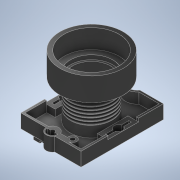
# Autodesk Inventor part: BASE DO BOTÃO
Saved by Autodesk Inventor 2022 (Build 260153000, 153)
## iProperties
Created: 2023-07-19
Part Number: BASE DO BOTÃO
Material: Acetal Resin, Black
Document SubType Name: Modeling
Designer: Usuário
Density: 1.425 g/cm^3
Appearance: Glossy - Black
Author: Usuário
Autodesk Inventor part; units mm, degrees
sketch "Sketch1" plane through (0, 0, 0) normal (0, 1, 0) x (-1, 0, 0)
  line L0 (0, 0) -> (30, 0)
  line L1 (30, 0) -> (30, -40)
  line L2 (30, -40) -> (0, -40)
  line L3 (0, -40) -> (0, 0)
  dimension "d0" = 30
  dimension "d1" = 40
  constraints: 8 end point, 2 parallel, 1 horizontal, 1 perpendicular
  measures "d0" distance of L1.end L2.end
  measures "d1" distance of L0.end L1.end
extrude "Extrusion1" add sketch "Sketch1" along normal blind 6.5
sketch "Sketch2" plane through (0, 0, 0) normal (0, -1, 0) x (1, 0, 0)
  circle A0 centre (-15, -20) radius 9
  line L0 (0, 0) -> (0, -40) projected
  line L1 (0, -40) -> (-30, -40) projected
  line L2 (0, 0) -> (0, -40) projected
  line L3 (0, -20) -> (-30, -20) construction
  line L4 (-30, -40) -> (-30, 0) projected
  line L5 (0, -40) -> (-30, -40) projected
  line L6 (-2.3, -14.5) -> (-2.3, -25.5) construction
  line L7 (-1.7, -14.5) -> (-2.9, -14.5)
  line L8 (-1.7, -25.5) -> (-2.9, -25.5)
  line L9 (-1.7, -14.5) -> (-1.7, -18.0921)
  line L10 (-1.7, -21.9079) -> (-1.7, -25.5)
  arc A1 (-2.9, -18.0921) -> (-2.9, -21.9079) centre (-2.3, -20) ccw
  arc A2 (-1.7, -21.9079) -> (-1.7, -18.0921) centre (-2.3, -20) ccw
  line L11 (-2.9, -14.5) -> (-2.9, -18.0921)
  line L12 (-2.9, -21.9079) -> (-2.9, -25.5)
  line L13 (-27.7, -14.5) -> (-27.7, -25.5) construction
  line L14 (-28.3, -14.5) -> (-27.1, -14.5)
  line L15 (-28.3, -25.5) -> (-27.1, -25.5)
  line L16 (-28.3, -14.5) -> (-28.3, -18.0921)
  line L17 (-28.3, -21.9079) -> (-28.3, -25.5)
  arc A3 (-27.1, -21.9079) -> (-27.1, -18.0921) centre (-27.7, -20) ccw
  arc A4 (-28.3, -18.0921) -> (-28.3, -21.9079) centre (-27.7, -20) ccw
  line L18 (-27.1, -14.5) -> (-27.1, -18.0921)
  line L19 (-27.1, -21.9079) -> (-27.1, -25.5)
  circle A5 centre (-1.5, -26.25) radius 0.75
  circle A6 centre (-1.5, -13.75) radius 0.75
  circle A7 centre (-28.5, -26.25) radius 0.75
  circle A8 centre (-28.5, -13.75) radius 0.75
  arc A9 (-11.063, -39) -> (-19.5, -40) centre (-15, -41.875) ccw
  line L20 (0, -39) -> (-11.063, -39)
  circle A10 centre (-23, -37) radius 1
  circle A11 centre (-7, -3) radius 1
  line L21 (-30, 0) -> (0, 0) projected
  arc A12 (-12.4019, 0) -> (-18, -1.5) centre (-15, -1.5) ccw
  line L22 (1.4111, 1.5) -> (-15, 1.5) construction
  line L23 (-17.5, -1.5) -> (-30, -1.5)
  line L24 (-15, -40) -> (-15, -4) construction
  arc A13 (-12.5, -1.5) -> (-17.5, -1.5) centre (-15, -1.5) ccw
  line L25 (-12.5, -1.5) -> (-17.5, -1.5)
  arc A14 (-16, -1.5) -> (-14, -1.5) centre (-15, -1.5) ccw
  circle A15 centre (-19, -5.5) radius 0.5
  line L26 (-30, 0) -> (0, 0) projected
  line L27 (-17.5981, 0) -> (-30, 0)
  line L28 (-30, 0) -> (-30, -1.5)
  point P0 (-19.5, -40)
  point P1 (-17, 0)
  point P2 (-13, 0)
  dimension "d4" = 18
  dimension "d5" = 0
  dimension "d8" = 2.3
  dimension "d9" = 11
  dimension "d10" = 5.5
  dimension "d13" = 5.5
  dimension "d14" = 5.5
  dimension "d15" = 2
  dimension "d16" = 1.2
  dimension "d17" = 3.5921
  dimension "d18" = 1.2
  dimension "d19" = 3.5921
  dimension "d20" = 2
  dimension "d21" = 1.5
  dimension "d22" = 1.5
  dimension "d24" = 1.5
  dimension "d25" = 1.5
  dimension "d29" = 1
  dimension "d30" = 2
  dimension "d31" = 7
  dimension "d32" = 3
  dimension "d33" = 2
  dimension "d34" = 7
  dimension "d35" = 3
  dimension "d36" = 6
  dimension "d37" = 1.5
  dimension "d38" = 3
  dimension "d39" = 0.5
  dimension "d40" = 2
  dimension "d41" = 1
  dimension "d42" = 19
  dimension "d43" = 4
  dimension "d122" = 1.5
  dimension "d123" = 1.5
  dimension "d124" = 1.7
  dimension "d125" = 1.4
  dimension "d126" = 1.7
  dimension "d127" = 1.4
  dimension "d128" = 0.75
  dimension "d129" = 6.25
  dimension "d130" = 0.75
  dimension "d131" = 5.5
  dimension "d132" = 5.5
  dimension "d136" = 1.5
  dimension "d137" = 1.2
  dimension "d138" = 2.3
  dimension "d139" = 2
  dimension "d140" = 2
  dimension "d141" = 1.2
  dimension "d142" = 11
  dimension "d143" = 1.5
  dimension "d144" = 1.7
  dimension "d145" = 1.7
  dimension "d146" = 1.4
  dimension "d147" = 6.25
  dimension "d148" = 6.25
  dimension "d151" = 6.25
  constraints: 44 end point, 18 point on circle, 16 centre point, 7 point on line, 6 parallel, 4 horizontal, 3 midpoint, 2 vertical, 1 coincident, 1 perpendicular, 1 tangent
  measures "d4" diameter of A0
  measures "d5" distance from line of L3 A0.centre
  measures "d8" distance from line of A1.centre L0
  measures "d9" distance of L6.start L6.end
  measures "d10" distance of L6.start A1.centre
  measures "d13" distance from line of L8 A1.centre
  measures "d14" distance from line of L7 A1.centre
  measures "d15" radius of A2
  measures "d16" distance between parallel lines of L12 L10
  measures "d17" distance of L10.start L8.start
  measures "d18" distance between parallel lines of L11 L9
  measures "d19" distance of L7.start L9.end
  measures "d20" radius of A1
  measures "d21" diameter of A5
  measures "d22" diameter of A6
  measures "d24" distance from line of L0 A5.centre
  measures "d25" distance from line of L0 A6.centre
  measures "d29" distance between parallel lines of L1 L20
  measures "d30" diameter of A10
  measures "d31" distance from line of A10.centre L4
  measures "d32" distance from line of A10.centre L1
  measures "d33" diameter of A11
  measures "d34" distance from line of L2 A11.centre
  measures "d35" distance from line of A11.centre L21
  measures "d36" diameter of A12
  measures "d37" distance between parallel lines of L21 L22
  measures "d38" distance between parallel lines of L22 L23
  measures "d39" radial gap between concentric circles of A12 A13
  measures "d40" diameter of A14
  measures "d41" diameter of A15
  measures "d42" distance from line of L0 A15.centre
  measures "d43" distance from line of L23 A15.centre
  measures "d122" distance from line of L4 A7.centre
  measures "d123" distance from line of L4 A8.centre
  measures "d124" distance from line of L3.start L10
  measures "d125" distance edge to line of A1 L12
  measures "d126" distance between parallel lines of L0 L9
  measures "d127" distance edge to line of A1 L11
  measures "d128" distance from line of L8 A5.centre
  measures "d129" vertical distance of A6.centre A1.centre
  measures "d130" distance from line of L7 A6.centre
  measures "d131" distance from line of L15 A3.centre
  measures "d132" distance from line of L14 A3.centre
  measures "d136" diameter of A7
  measures "d137" distance between parallel lines of L19 L17
  measures "d138" distance from line of L4 A3.centre
  measures "d139" radius of A3
  measures "d140" radius of A4
  measures "d141" distance between parallel lines of L16 L18
  measures "d142" distance from line of L13.end L14
  measures "d143" diameter of A8
  measures "d144" distance between parallel lines of L4 L17
  measures "d145" distance between parallel lines of L4 L16
  measures "d146" distance edge to line of A3 L19
  measures "d147" vertical distance of A8.centre A3.centre
  measures "d148" vertical distance of A7.centre A3.centre
  measures "d151" vertical distance of A5.centre A1.centre
extrude "Extrusion2" cut sketch "Sketch2" against normal blind 6.5 contours A0 | L0 L1 A9 L20 | A13 L25 L21 | L21 A13 | A12 L23 L4 L21 | A14 L25 | L9 A2 L10 L8 L12 A1 L11 L7 | L14 L18 A3 L19 L15 L17 A4 L16 | A10 | A11
extrude "Extrusion3" add sketch "Sketch2" along normal blind 0.5 contours A15
extrude "Extrusion4" add sketch "Sketch2" against normal up to surface (6.5 mm away) contours L21 A13 A12
sketch "Sketch3" plane through (0, 6.5, 0) normal (0, 1, 0) x (1, 0, 0)
  line L0 (0, 20) -> (-30, 20) construction
  line L1 (0, 12.75) -> (-5, 12.75)
  line L2 (0, 27.25) -> (-5, 27.25)
  line L3 (0, 0) -> (0, 39)
  line L4 (-5, 12.75) -> (-5, 27.25)
  line L5 (-15, 40) -> (-15, 4) construction
  line L6 (-30, 12.75) -> (-25, 12.75)
  line L7 (-30, 27.25) -> (-25, 27.25)
  line L8 (-25, 12.75) -> (-25, 27.25)
  line L9 (-30, 40) -> (-30, 1.5)
  arc A0 (-27.1, 18.0921) -> (-27.1, 21.9079) centre (-27.7, 20) ccw projected
  line L10 (-12.4019, 0) -> (0, 0) projected
  line L11 (0, 0) -> (0, 39) projected
  line L12 (0, 39) -> (-11.063, 39) projected
  arc A1 (-19.5, 40) -> (-11.063, 39) centre (-15, 41.875) ccw projected
  line L13 (-19.5, 40) -> (-30, 40) projected
  line L14 (-30, 40) -> (-30, 1.5) projected
  line L15 (-30, 1.5) -> (-18, 1.5) projected
  arc A2 (-18, 1.5) -> (-12.4019, 0) centre (-15, 1.5) ccw projected
  line L16 (-28.3, 25.5) -> (-27.1, 25.5) projected
  line L17 (-27.1, 25.5) -> (-27.1, 21.9079) projected
  arc A3 (-27.1, 18.0921) -> (-27.1, 21.9079) centre (-27.7, 20) ccw projected
  line L18 (-27.1, 18.0921) -> (-27.1, 14.5) projected
  line L19 (-27.1, 14.5) -> (-28.3, 14.5) projected
  line L20 (-28.3, 14.5) -> (-28.3, 18.0921) projected
  arc A4 (-28.3, 21.9079) -> (-28.3, 18.0921) centre (-27.7, 20) ccw projected
  line L21 (-28.3, 21.9079) -> (-28.3, 25.5) projected
  circle A5 centre (-23, 37) radius 1 projected
  line L22 (-1.7, 14.5) -> (-2.9, 14.5) projected
  line L23 (-2.9, 14.5) -> (-2.9, 18.0921) projected
  arc A6 (-2.9, 21.9079) -> (-2.9, 18.0921) centre (-2.3, 20) ccw projected
  line L24 (-2.9, 21.9079) -> (-2.9, 25.5) projected
  line L25 (-2.9, 25.5) -> (-1.7, 25.5) projected
  line L26 (-1.7, 25.5) -> (-1.7, 21.9079) projected
  arc A7 (-1.7, 18.0921) -> (-1.7, 21.9079) centre (-2.3, 20) ccw projected
  line L27 (-1.7, 18.0921) -> (-1.7, 14.5) projected
  circle A8 centre (-15, 20) radius 9 projected
  circle A9 centre (-7, 3) radius 1 projected
  arc A10 (-17.5, 1.5) -> (-12.5, 1.5) centre (-15, 1.5) ccw projected
  line L28 (-17.5, 1.5) -> (-16, 1.5) projected
  arc A11 (-14, 1.5) -> (-16, 1.5) centre (-15, 1.5) ccw projected
  line L29 (-14, 1.5) -> (-12.5, 1.5) projected
  dimension "d50" = 7.25
  dimension "d51" = 7.25
  dimension "d52" = 5
  dimension "d149" = 7.25
  dimension "d150" = 7.25
  constraints: 16 end point, 4 symmetric about line, 2 parallel
  measures "d50" distance between parallel lines of L0 L1
  measures "d51" distance between parallel lines of L0 L2
  measures "d52" distance between parallel lines of L3 L4
  measures "d149" distance from line of L7 A0.centre
  measures "d150" distance from line of L6 A0.centre
extrude "Extrusion5" cut sketch "Sketch2" against normal blind 1 contours A5 | A6 | A7 | A8
extrude "Extrusion6" cut sketch "Sketch3" against normal blind 1.6 contours L1 L4 L2 L3 | L9 L7 L8 L6 | L18 L19 L20 A4 L21 L16 L17 A0 | L22 L23 A6 L24 L25 L26 A7 L27
sketch "Sketch4" plane through (0, 6.5, 0) normal (0, 1, 0) x (1, 0, 0)
  circle A0 centre (-23, 37) radius 1 projected
  circle A1 centre (-23, 37) radius 2.9845
  arc A2 (-17.5, 1.5) -> (-12.5, 1.5) centre (-15, 1.5) ccw
  line L0 (-17.5, 1.5) -> (-16, 1.5) projected
  arc A3 (-16, 1.5) -> (-14, 1.5) centre (-15, 1.5) ccw projected
  line L1 (-14, 1.5) -> (-12.5, 1.5) projected
  circle A4 centre (-7, 3) radius 1 projected
  circle A5 centre (-15, 20) radius 9 projected
  circle A6 centre (-23, 37) radius 1 projected
  line L2 (0, 12.75) -> (-5, 12.75) projected
  line L3 (-5, 12.75) -> (-5, 27.25) projected
  line L4 (-5, 27.25) -> (0, 27.25) projected
  line L5 (0, 27.25) -> (0, 39) projected
  line L6 (0, 39) -> (-11.063, 39) projected
  arc A7 (-11.063, 39) -> (-19.5, 40) centre (-15, 41.875) ccw projected
  line L7 (-19.5, 40) -> (-30, 40) projected
  line L8 (-30, 40) -> (-30, 27.25) projected
  line L9 (-30, 27.25) -> (-25, 27.25) projected
  line L10 (-25, 27.25) -> (-25, 12.75) projected
  line L11 (-25, 12.75) -> (-30, 12.75) projected
  line L12 (-30, 12.75) -> (-30, 1.5) projected
  line L13 (-30, 1.5) -> (-18, 1.5) projected
  arc A8 (-12.4019, 0) -> (-18, 1.5) centre (-15, 1.5) ccw projected
  line L14 (-12.4019, 0) -> (0, 0) projected
  line L15 (0, 0) -> (0, 12.75) projected
  line L16 (-29, 39) -> (-20.1235, 39)
  arc A9 (-20.1235, 39) -> (-10.5841, 38) centre (-15, 41.875) ccw
  line L17 (-10.5841, 38) -> (-1, 38)
  line L18 (-1, 38) -> (-1, 27.25)
  line L19 (-1, 12.75) -> (-1, 1)
  line L20 (-16.7321, 2.5) -> (-29, 2.5)
  line L21 (-29, 2.5) -> (-29, 12.75)
  line L22 (-29, 27.25) -> (-29, 39)
  circle A10 centre (-7, 3) radius 2.0133
  line L23 (-1, 1) -> (-7.2306, 1)
  arc A11 (-17.5, 1.5) -> (-12.5, 1.5) centre (-15, 1.5) ccw projected
  line L24 (-17.5, 1.5) -> (-17.5, 3.1583)
  line L25 (-12.5, 1.5) -> (-12.5, 2.5)
  line L26 (-12.5, 2.5) -> (-8.9502, 2.5)
  arc A12 (-17.5, 1.5) -> (-12.5, 1.5) centre (-15, 1.5) ccw projected
  line L27 (-17.5, 1.5) -> (-16, 1.5) projected
  arc A13 (-14, 1.5) -> (-16, 1.5) centre (-15, 1.5) ccw projected
  line L28 (-14, 1.5) -> (-12.5, 1.5) projected
  circle A14 centre (-7, 3) radius 1 projected
  circle A15 centre (-15, 20) radius 9 projected
  circle A16 centre (-23, 37) radius 1 projected
  line L29 (0, 12.75) -> (-5, 12.75) projected
  line L30 (-5, 12.75) -> (-5, 27.25) projected
  line L31 (-5, 27.25) -> (0, 27.25) projected
  line L32 (0, 27.25) -> (0, 39) projected
  line L33 (0, 39) -> (-11.063, 39) projected
  arc A17 (-19.5, 40) -> (-11.063, 39) centre (-15, 41.875) ccw projected
  line L34 (-19.5, 40) -> (-30, 40) projected
  line L35 (-30, 40) -> (-30, 27.25) projected
  line L36 (-30, 27.25) -> (-25, 27.25) projected
  line L37 (-25, 27.25) -> (-25, 12.75) projected
  line L38 (-25, 12.75) -> (-30, 12.75) projected
  line L39 (-30, 12.75) -> (-30, 1.5) projected
  line L40 (-30, 1.5) -> (-18, 1.5) projected
  arc A18 (-18, 1.5) -> (-12.4019, 0) centre (-15, 1.5) ccw projected
  line L41 (-12.4019, 0) -> (0, 0) projected
  line L42 (0, 0) -> (0, 12.75) projected
  circle A19 centre (-15, 20) radius 10
  point P0 (-29, 12)
  point P1 (-29, 28)
  point P2 (-20.7847, 39)
  point P3 (-25.2153, 39)
  point P4 (-25, 20)
  point P5 (-5, 20)
  point P6 (-17.8284, 2.5)
  point P7 (-12.1716, 2.5)
  point P8 (-6.7694, 1)
  dimension "d57" = 1
  dimension "d60" = 20
  constraints: 22 end point, 11 centre point, 6 point on circle, 6 point on line, 1 coincident, 1 perpendicular, 1 vertical, 4 other
  measures "d57" distance between parallel lines of L7 L16
  measures "d60" diameter of A19
extrude "Extrusion7" add sketch "Sketch4" along normal blind 13 contours A19
sketch "Sketch6" plane through (-15, 19.5, -20) normal (0, 1, 0) x (1, 0, 0)
  circle A0 centre (0, 0) radius 15
  circle A1 centre (0, 0) radius 10 projected
  circle A2 centre (0, 0) radius 13
  point P0 (15, -20)
  dimension "d63" = 30
  dimension "d152" = 2
  constraints: 2 centre point
  measures "d63" diameter of A0
  measures "d152" radial gap between concentric circles of A0 A2
extrude "Extrusion8" add sketch "Sketch6" along normal blind 2 contours A0 | A2
ref_plane "Work Plane2" through (-15, 32.5, -20) normal (0, 1, 0) x (1, 0, 0)
ref_plane "Work Plane1" through (-15, 25.5, -20) normal (0, 1, 0) x (1, 0, 0)
ref_plane "Work Plane3" through (-15, 25.5, -20) normal (0, 1, 0) x (1, 0, 0)
thread "Thread1" size "M20x1.5" standard "Din Taper" length 8.5
extrude "Extrusion13" cut sketch "Sketch4" against normal blind 5 contours A1 L16 A9 L17 L18 L4 L3 A19 L10 L9 L22 | A19 L3 L2 L19 L23 A10 L26 A8 L20 L21 L11 L10
sketch "Sketch11" plane through (0, 0, 0) normal (0, -1, 0) x (1, 0, 0)
  line L0 (-11.063, -39) -> (-8.063, -39)
  line L1 (-8.063, -39) -> (-8.063, -37)
  line L2 (-8.063, -37) -> (-11.063, -37)
  line L3 (-11.063, -37) -> (-11.063, -39)
  line L4 (-8.063, -39) -> (-5.063, -39)
  line L5 (-5.063, -39) -> (-5.063, -37)
  line L6 (-5.063, -37) -> (-8.063, -37)
  line L7 (-8.063, -37) -> (-8.063, -39)
  line L8 (-23.987, -3.5068) -> (-20.987, -3.5068)
  line L9 (-20.987, -3.5068) -> (-20.987, -1.5068)
  line L10 (-20.987, -1.5068) -> (-23.987, -1.5068)
  line L11 (-23.987, -1.5068) -> (-23.987, -3.5068)
  line L12 (-20.987, -1.5068) -> (-20.987, -3.5068)
  line L13 (-20.987, -3.5068) -> (-17.987, -3.5068)
  line L14 (-17.987, -3.5068) -> (-17.987, -1.5068)
  line L15 (-17.987, -1.5068) -> (-20.987, -1.5068)
  point P0 (0, 0)
  dimension "d98" = 3
  dimension "d99" = 2
  dimension "d100" = 3
  dimension "d101" = 2
  dimension "d106" = 3
  dimension "d107" = 2
  dimension "d108" = 3
  dimension "d109" = 2
  constraints: 32 end point, 8 parallel, 4 horizontal, 4 perpendicular
  measures "d98" distance of L2.end L1.end
  measures "d99" distance of L1.end L0.end
  measures "d100" distance of L7.start L5.end
  measures "d101" distance of L5.end L4.end
  measures "d106" distance of L10.end L9.end
  measures "d107" distance of L9.end L8.end
  measures "d108" distance of L12.start L14.end
  measures "d109" distance of L14.end L13.end
extrude "Extrusion14" add sketch "Sketch11" along normal blind 0.5 contours L3 L2 L1 L0
extrude "Extrusion15" add sketch "Sketch11" along normal blind 1.5 contours L1 L6 L5 L4
extrude "Extrusion16" add sketch "Sketch11" along normal blind 0.5 contours L9 L15 L14 L13
extrude "Extrusion17" add sketch "Sketch11" along normal blind 1.5 contours L11 L10 L9 L8
sketch "Sketch12" plane through (0, -0.5, 0) normal (0, -1, 0) x (1, 0, 0)
  line L0 (-18.6214, -1.6631) -> (-18.6214, -3.4135) construction
  line L1 (-18.6214, -3.4135) -> (-20.1263, -3.4135) construction
  line L2 (-20.1263, -3.4135) -> (-20.1263, -1.6631) construction
  line L3 (-20.1263, -1.6631) -> (-18.6214, -1.6631) construction
  line L4 (-10.4155, -38.734) -> (-10.4155, -36.9836) construction
  line L5 (-10.4155, -36.9836) -> (-8.9106, -36.9836) construction
  line L6 (-8.9106, -36.9836) -> (-8.9106, -38.734) construction
  line L7 (-8.9106, -38.734) -> (-10.4155, -38.734) construction
  line L8 (-20.1263, -2.6222) -> (-20.1263, -1.8904)
  line L9 (-20.1263, -1.8904) -> (-19.9731, -1.8904)
  line L10 (-19.9731, -1.8904) -> (-19.9731, -2.1627)
  line L11 (-19.9731, -2.1627) -> (-18.9678, -2.1627)
  line L12 (-18.9678, -2.1627) -> (-18.9678, -1.8904)
  line L13 (-18.9678, -1.8904) -> (-18.8305, -1.8904)
  spline S0 degree 2 poles (-18.8305, -1.8904) (-18.8305, -2.0448) (-18.743, -2.1906) (-18.6214, -2.2004) knots 0 0 0 1 2 2 2
  line L14 (-18.6214, -2.2004) -> (-18.6214, -2.356)
  line L15 (-18.6214, -2.356) -> (-19.9731, -2.356)
  line L16 (-19.9731, -2.356) -> (-19.9731, -2.6222)
  line L17 (-19.9731, -2.6222) -> (-20.1263, -2.6222)
  line L18 (-20.1263, -3.2202) -> (-20.1263, -2.9795)
  line L19 (-20.1263, -2.9795) -> (-19.8394, -2.9795)
  line L20 (-19.8394, -2.9795) -> (-19.8394, -3.2202)
  line L21 (-19.8394, -3.2202) -> (-20.1263, -3.2202)
  line L22 (-8.8839, -37.6996) -> (-8.8839, -38.6246)
  line L23 (-8.8839, -38.6246) -> (-9.0966, -38.6246)
  spline S1 degree 2 poles (-9.0966, -38.6246) (-9.1902, -38.5249) (-9.364, -38.3475) (-9.4576, -38.2624) knots 0 0 0 1 2 2 2
  spline S2 degree 2 poles (-9.4576, -38.2624) (-9.646, -38.091) (-9.8721, -37.9658) (-9.9924, -37.9658) knots 0 0 0 1 2 2 2
  spline S3 degree 2 poles (-9.9924, -37.9658) (-10.0557, -37.9658) (-10.1505, -38.0047) (-10.1809, -38.0399) knots 0 0 0 1 2 2 2
  spline S4 degree 2 poles (-10.1809, -38.0399) (-10.2112, -38.0752) (-10.2416, -38.1676) (-10.2416, -38.2235) knots 0 0 0 1 2 2 2
  spline S5 degree 2 poles (-10.2416, -38.2235) (-10.2416, -38.277) (-10.2149, -38.3864) (-10.1942, -38.4362) knots 0 0 0 1 2 2 2
  spline S6 degree 2 poles (-10.1942, -38.4362) (-10.1772, -38.4787) (-10.1286, -38.5578) (-10.1116, -38.5821) knots 0 0 0 1 2 2 2
  line L24 (-10.1116, -38.5821) -> (-10.1116, -38.593)
  line L25 (-10.1116, -38.593) -> (-10.3255, -38.593)
  spline S7 degree 2 poles (-10.3255, -38.593) (-10.3559, -38.531) (-10.4155, -38.3086) (-10.4155, -38.2089) knots 0 0 0 1 2 2 2
  spline S8 degree 2 poles (-10.4155, -38.2089) (-10.4155, -37.9986) (-10.193, -37.7616) (-10.0034, -37.7616) knots 0 0 0 1 2 2 2
  spline S9 degree 2 poles (-10.0034, -37.7616) (-9.9146, -37.7616) (-9.7663, -37.8029) (-9.7031, -37.8394) knots 0 0 0 1 2 2 2
  spline S10 degree 2 poles (-9.7031, -37.8394) (-9.6375, -37.8758) (-9.5086, -37.9816) (-9.4467, -38.0399) knots 0 0 0 1 2 2 2
  spline S11 degree 2 poles (-9.4467, -38.0399) (-9.3433, -38.1347) (-9.1221, -38.3669) (-9.0577, -38.4362) knots 0 0 0 1 2 2 2
  line L26 (-9.0577, -38.4362) -> (-9.0577, -37.6996)
  line L27 (-9.0577, -37.6996) -> (-8.8839, -37.6996)
  line L28 (-8.8839, -37.1769) -> (-8.8839, -37.4176)
  line L29 (-8.8839, -37.4176) -> (-9.1707, -37.4176)
  line L30 (-9.1707, -37.4176) -> (-9.1707, -37.1769)
  line L31 (-9.1707, -37.1769) -> (-8.8839, -37.1769)
  point P0 (0, 0)
  constraints: 4 other
sketch "Sketch13" plane through (0, -1.5, 0) normal (0, -1, 0) x (1, 0, 0)
  line L0 (-21.6073, -1.6939) -> (-21.6073, -3.4443) construction
  line L1 (-21.6073, -3.4443) -> (-23.1705, -3.4443) construction
  line L2 (-23.1705, -3.4443) -> (-23.1705, -1.6939) construction
  line L3 (-23.1705, -1.6939) -> (-21.6073, -1.6939) construction
  line L4 (-7.1447, -38.6959) -> (-7.1447, -36.9455) construction
  line L5 (-7.1447, -36.9455) -> (-5.5815, -36.9455) construction
  line L6 (-5.5815, -36.9455) -> (-5.5815, -38.6959) construction
  line L7 (-5.5815, -38.6959) -> (-7.1447, -38.6959) construction
  line L8 (-6.1601, -37.6213) -> (-6.1601, -37.8)
  line L9 (-6.1601, -37.8) -> (-5.6447, -37.8)
  line L10 (-5.6447, -37.8) -> (-5.6447, -37.9933)
  line L11 (-5.6447, -37.9933) -> (-6.1601, -37.9933)
  line L12 (-6.1601, -37.9933) -> (-6.1601, -38.6558)
  line L13 (-6.1601, -38.6558) -> (-6.3716, -38.6558)
  line L14 (-6.3716, -38.6558) -> (-7.1447, -37.9848)
  line L15 (-7.1447, -37.9848) -> (-7.1447, -37.8)
  line L16 (-7.1447, -37.8) -> (-6.3218, -37.8)
  line L17 (-6.3218, -37.8) -> (-6.3218, -37.6213)
  line L18 (-6.3218, -37.6213) -> (-6.1601, -37.6213)
  line L19 (-6.3218, -37.9933) -> (-6.9077, -37.9933)
  line L20 (-6.9077, -37.9933) -> (-6.3218, -38.4978)
  line L21 (-6.3218, -38.4978) -> (-6.3218, -37.9933)
  line L22 (-5.6447, -37.1388) -> (-5.6447, -37.3794)
  line L23 (-5.6447, -37.3794) -> (-5.9316, -37.3794)
  line L24 (-5.9316, -37.3794) -> (-5.9316, -37.1388)
  line L25 (-5.9316, -37.1388) -> (-5.6447, -37.1388)
  spline S0 degree 2 poles (-21.7811, -2.2081) (-21.7811, -2.1534) (-21.8079, -2.0452) (-21.8285, -1.993) knots 0 0 0 1 2 2 2
  spline S1 degree 2 poles (-21.8285, -1.993) (-21.8492, -1.9443) (-21.893, -1.8726) (-21.9124, -1.8447) knots 0 0 0 1 2 2 2
  line L26 (-21.9124, -1.8447) -> (-21.9124, -1.8325)
  line L27 (-21.9124, -1.8325) -> (-21.6997, -1.8325)
  spline S2 degree 2 poles (-21.6997, -1.8325) (-21.6644, -1.8982) (-21.6073, -2.123) (-21.6073, -2.2239) knots 0 0 0 1 2 2 2
  spline S3 degree 2 poles (-21.6073, -2.2239) (-21.6073, -2.326) (-21.6486, -2.478) (-21.6924, -2.54) knots 0 0 0 1 2 2 2
  spline S4 degree 2 poles (-21.6924, -2.54) (-21.7398, -2.6056) (-21.8772, -2.6737) (-21.9695, -2.6737) knots 0 0 0 1 2 2 2
  spline S5 degree 2 poles (-21.9695, -2.6737) (-22.0935, -2.6737) (-22.2807, -2.5108) (-22.305, -2.3965) knots 0 0 0 1 2 2 2
  line L28 (-22.305, -2.3965) -> (-22.3196, -2.3965)
  spline S6 degree 2 poles (-22.3196, -2.3965) (-22.3293, -2.4439) (-22.3731, -2.5521) (-22.4169, -2.5983) knots 0 0 0 1 2 2 2
  spline S7 degree 2 poles (-22.4169, -2.5983) (-22.4594, -2.6445) (-22.5956, -2.7029) (-22.694, -2.7029) knots 0 0 0 1 2 2 2
  spline S8 degree 2 poles (-22.694, -2.7029) (-22.7949, -2.7029) (-22.9663, -2.6336) (-23.0319, -2.5704) knots 0 0 0 1 2 2 2
  spline S9 degree 2 poles (-23.0319, -2.5704) (-23.1, -2.5047) (-23.1705, -2.3187) (-23.1705, -2.2008) knots 0 0 0 1 2 2 2
  spline S10 degree 2 poles (-23.1705, -2.2008) (-23.1705, -2.0878) (-23.1158, -1.8665) (-23.0781, -1.7912) knots 0 0 0 1 2 2 2
  line L29 (-23.0781, -1.7912) -> (-22.8654, -1.7912)
  line L30 (-22.8654, -1.7912) -> (-22.8654, -1.8058)
  spline S11 degree 2 poles (-22.8654, -1.8058) (-22.9116, -1.869) (-22.9967, -2.0829) (-22.9967, -2.1887) knots 0 0 0 1 2 2 2
  spline S12 degree 2 poles (-22.9967, -2.1887) (-22.9967, -2.2507) (-22.9578, -2.3746) (-22.9128, -2.416) knots 0 0 0 1 2 2 2
  spline S13 degree 2 poles (-22.9128, -2.416) (-22.8678, -2.4561) (-22.7609, -2.4986) (-22.6794, -2.4986) knots 0 0 0 1 2 2 2
  spline S14 degree 2 poles (-22.6794, -2.4986) (-22.598, -2.4986) (-22.4922, -2.4512) (-22.4618, -2.4087) knots 0 0 0 1 2 2 2
  spline S15 degree 2 poles (-22.4618, -2.4087) (-22.4315, -2.3661) (-22.4084, -2.2507) (-22.4084, -2.1826) knots 0 0 0 1 2 2 2
  line L31 (-22.4084, -2.1826) -> (-22.4084, -2.0975)
  line L32 (-22.4084, -2.0975) -> (-22.2418, -2.0975)
  line L33 (-22.2418, -2.0975) -> (-22.2418, -2.1644)
  spline S16 degree 2 poles (-22.2418, -2.1644) (-22.2418, -2.2993) (-22.113, -2.4695) (-21.9902, -2.4695) knots 0 0 0 1 2 2 2
  spline S17 degree 2 poles (-21.9902, -2.4695) (-21.9331, -2.4695) (-21.8516, -2.4257) (-21.8273, -2.3905) knots 0 0 0 1 2 2 2
  spline S18 degree 2 poles (-21.8273, -2.3905) (-21.8018, -2.3528) (-21.7811, -2.2604) (-21.7811, -2.2081) knots 0 0 0 1 2 2 2
  line L34 (-23.1389, -3.2511) -> (-23.1389, -3.0104)
  line L35 (-23.1389, -3.0104) -> (-22.852, -3.0104)
  line L36 (-22.852, -3.0104) -> (-22.852, -3.2511)
  line L37 (-22.852, -3.2511) -> (-23.1389, -3.2511)
  point P0 (0, 0)
  constraints: 4 other
emboss "Emboss1" sketch "Sketch12" operation cut depth 0.1 direction (0, 1, 0) contours L8 L9 L10 L11 L12 L13 S0 L14 L15 L16 L17 | L18 L19 L20 L21
emboss "Emboss2" sketch "Sketch12" operation cut depth 0.1 direction (0, 1, 0) contours L22 L23 S1 S2 S3 S4 S5 S6 L24 L25 S7 S8 S9 S10 S11 L26 L27 | L28 L29 L30 L31
emboss "Emboss3" sketch "Sketch13" operation cut depth 0.1 direction (0, 1, 0) contours L8 L9 L10 L11 L12 L13 L14 L15 L16 L17 L18 | L22 L23 L24 L25
emboss "Emboss4" sketch "Sketch13" operation cut depth 0.1 direction (0, 1, 0) contours S0 S1 L26 L27 S2 S3 S4 S5 L28 S6 S7 S8 S9 S10 L29 L30 S11 S12 S13 S14 S15 L31 L32 L33 S16 S17 S18 | L34 L35 L36 L37
sketch "Sketch14" plane through (-15, 21.5, -20) normal (0, 1, 0) x (1, 0, 0)
  circle A0 centre (0, 0) radius 15 projected
  circle A1 centre (0, 0) radius 13 projected
  point P0 (15, -20)
extrude "Extrusion18" add sketch "Sketch14" along normal blind 9
ref_plane "Work Plane4" through (0, 7, 0) normal (0, -1, 0) x (1, 0, 0)
sketch "Sketch15" plane through (0, 7, 0) normal (0, -1, 0) x (1, 0, 0)
  circle A0 centre (-15, -20) radius 9 projected
  circle A1 centre (-15, -20) radius 11
  circle A2 centre (-15, -20) radius 11
  circle A3 centre (-15, -20) radius 7
  point P0 (0, 0)
  dimension "d156" = 2
  dimension "d157" = 2
  dimension "d158" = 2
  constraints: 3 centre point
  measures "d156" radial gap between concentric circles of A0 A1
  measures "d157" radial gap between concentric circles of A0 A2
  measures "d158" radial gap between concentric circles of A0 A3
extrude "Extrusion19" add sketch "Sketch15" against normal blind 1 contours A0
equation "\"d123\" = d122"
body "Solid1"
